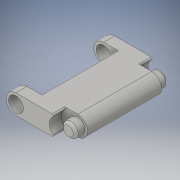
# Autodesk Inventor part: TrackDisplayStrapSegment
Saved by Autodesk Inventor 2016 (Build 200138000, 138)
## iProperties
Created: 2016-05-05
Part Number: TrackDisplayStrapSegment
Material: Generic
Document SubType Name: Modeling
Designer: xdlea
Density: 1 g/cm^3
Appearance: Default
Author: xdlea
Autodesk Inventor part; units mm, degrees
ref_plane "YZ Plane" through (0, 0, 0) normal (1, 0, 0) x (0, 1, 0)
ref_plane "XZ Plane" through (0, 0, 0) normal (0, 1, 0) x (-1, 0, 0)
ref_plane "XY Plane" through (0, 0, 0) normal (0, 0, 1) x (1, 0, 0)
sketch "Sketch1" plane through (0, 0, 0) normal (0, 0, 1) x (1, 0, 0)
  circle A0 centre (-6.35, 0) radius 1.905
  circle A1 centre (6.35, 0) radius 1.87325
  arc A2 (-6.35, 2.54) -> (-6.35, -2.54) centre (-6.35, 0) ccw
  line L0 (-6.35, 2.54) -> (4.7625, 2.54)
  line L1 (0, 3.556) -> (0, -3.556) construction
  line L2 (-12.446, 0) -> (12.446, 0) construction
  line L3 (-6.35, -2.54) -> (4.7625, -2.54)
  arc A3 (-3.453414, -2.54) -> (-3.453414, 2.54) centre (-4.7625, 0) ccw
  arc A4 (6.35, -2.54) -> (6.35, 2.54) centre (6.35, 0) ccw
  line L4 (4.7625, 2.54) -> (6.35, 2.54)
  line L5 (4.7625, -2.54) -> (6.35, -2.54)
  arc A5 (4.7625, 2.54) -> (4.7625, -2.54) centre (4.7625, 0) ccw
  dimension "d2" = 3.81
  dimension "d3" = 3.7465
  dimension "d5" = 5.08
  dimension "d6" = 12.7
  dimension "d16" = 1.5875
  dimension "d17" = 2.8575
  dimension "d18" = 1.5875
  constraints: 8 end point, 8 point on circle, 7 tangent, 6 centre point, 4 point on line, 2 coincident, 2 horizontal, 1 horizontal alignment, 1 symmetric about line, 1 vertical alignment
  measures "d2" diameter of A0
  measures "d3" diameter of A1
  measures "d5" distance between parallel lines of L3 L0
  measures "d6" distance of A1.centre A0.centre
  measures "d16" distance of A3.centre A0.centre
  measures "d17" radius of A3
  measures "d18" distance of A1.centre A5.centre
sketch "Sketch1 outline for Extrusion1" plane through (0, 0, 0) normal (0, 0, 1) x (1, 0, 0)
  arc A0 (4.7625, -2.54) -> (4.7625, 2.54) centre (4.7625, 0) cw
  line L0 (4.7625, 2.54) -> (-6.35, 2.54)
  arc A1 (-6.35, 2.54) -> (-6.35, -2.54) centre (-6.35, 0) ccw
  line L1 (-6.35, -2.54) -> (4.7625, -2.54)
  circle A2 centre (-6.35, 0) radius 1.905
extrude "Extrusion1" add sketch "Sketch1 outline for Extrusion1" along normal mid plane 25.4
sketch "Sketch1 outline for Extrusion2" plane through (0, 0, 0) normal (0, 0, 1) x (1, 0, 0)
  arc A0 (4.7625, 2.54) -> (4.7625, -2.54) centre (4.7625, 0) ccw
  line L0 (6.35, 2.54) -> (4.7625, 2.54)
  line L1 (4.7625, -2.54) -> (6.35, -2.54)
  arc A1 (6.35, -2.54) -> (6.35, 2.54) centre (6.35, 0) ccw
  circle A2 centre (6.35, 0) radius 1.87325
extrude "Extrusion2" add sketch "Sketch1 outline for Extrusion2" along normal mid plane 19.05
sketch "Sketch1 outline for Extrusion3" plane through (0, 0, 0) normal (0, 0, 1) x (1, 0, 0)
  line L0 (-3.453414, 2.54) -> (-6.35, 2.54)
  arc A0 (-3.453414, -2.54) -> (-3.453414, 2.54) centre (-4.7625, 0) ccw
  arc A1 (-6.35, 2.54) -> (-6.35, -2.54) centre (-6.35, 0) ccw
  line L1 (-6.35, -2.54) -> (-3.453414, -2.54)
  circle A2 centre (-6.35, 0) radius 1.905
extrude "Extrusion3" cut sketch "Sketch1 outline for Extrusion3" along normal mid plane 19.685
sketch "Sketch1 outline for Extrusion4" plane through (0, 0, 0) normal (0, 0, 1) x (1, 0, 0)
  circle A0 centre (6.35, 0) radius 1.87325
extrude "Extrusion4" add sketch "Sketch1 outline for Extrusion4" along normal mid plane 23.8125
chamfer "Chamfer1" distance 0.635 angle 45 2 edges at (4.4768, 0, 11.9062) (4.4768, 0, -11.9062)
fillet "Fillet1" radius 0.3175 6 edges at (-3.4534, 2.54, 0) (-3.4534, -2.54, 0) (4.7625, 2.54, 11.1125) (4.7625, 2.54, -11.1125) (4.7625, -2.54, 11.1125) (4.7625, -2.54, -11.1125)
equation "\"d18\" = d16"
body "Solid1"
